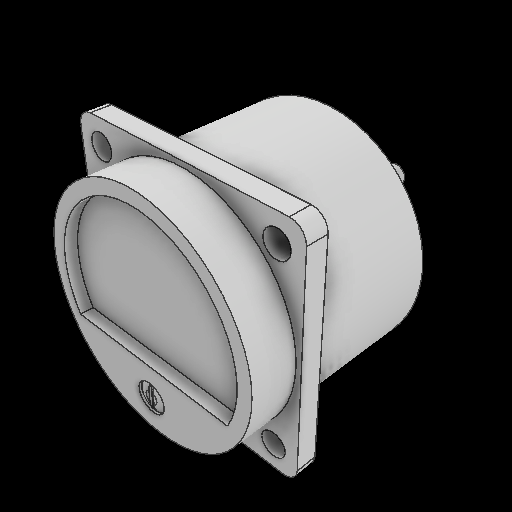
# Autodesk Inventor part: BaomanACPanelMountMeter
Saved by Autodesk Inventor 2025.2 (Build 292293000, 293)
## iProperties
Created: 2026-05-14
Part Number: BaomanACPanelMountMeter
Material: Generic
Document SubType Name: Modeling
Designer: valer
Density: 1 g/cm^3
Appearance: Default
Author: valer
Autodesk Inventor part; units mm, degrees
ref_plane "YZ Plane" through (0, 0, 0) normal (1, 0, 0) x (0, 1, 0)
ref_plane "XZ Plane" through (0, 0, 0) normal (0, 1, 0) x (-1, 0, 0)
ref_plane "XY Plane" through (0, 0, 0) normal (0, 0, 1) x (1, 0, 0)
sketch "Base" plane through (0, 0, 0) normal (0, 0, 1) x (1, 0, 0)
  line L0 (-23.5, -23.5) -> (23.5, -23.5)
  line L1 (23.5, -23.5) -> (23.5, 23.5)
  line L2 (23.5, 23.5) -> (-23.5, 23.5)
  line L3 (-23.5, 23.5) -> (-23.5, -23.5)
  line L4 (-23.5, -23.5) -> (23.5, 23.5) construction
  line L5 (23.5, -23.5) -> (-23.5, 23.5) construction
  point P0 (0, 0)
  dimension "d0" = 47
  constraints: 12 end point, 2 midpoint, 2 parallel, 2 perpendicular, 1 horizontal
  measures "d0" distance of L2.end L0.start
extrude "BaseFeature" add sketch "Base" along normal blind 4
fillet "FilletsFeature" radius 3 4 edges at (-23.5, -23.5, 2) (-23.5, 23.5, 2) (23.5, -23.5, 2) (23.5, 23.5, 2)
sketch "Front" plane through (0, 0, 4) normal (0, 0, 1) x (1, 0, 0)
  circle A0 centre (0, 0) radius 22.5
  dimension "d4" = 45
  constraints: 1 centre point, 1 coincident
  measures "d4" diameter of A0
extrude "FrontFeature" add sketch "Front" along normal blind 8.5
sketch "Screen" plane through (0, 0, 12.5) normal (0, 0, 1) x (1, 0, 0)
  circle A0 centre (0, 0) radius 19.7
  circle A1 centre (0, 0) radius 22.5 projected
  line L0 (-17.575, -8.9) -> (17.575, -8.9)
  line L1 (0, -8.9) -> (0, -19.7) construction
  dimension "d7" = 2.8
  dimension "d8" = 10.8
  constraints: 4 end point, 3 point on circle, 1 centre point, 1 coincident, 1 horizontal, 1 midpoint, 1 vertical
  measures "d7" radial gap between concentric circles of A1 A0
  measures "d8" distance of L1.start L1.end
extrude "ScreenFEature" cut sketch "Screen" against normal blind 2.5 contours A0 L0 picked at (4.7799, 0.8366)
sketch "ScrewHole" plane through (0, 0, 12.5) normal (0, 0, 1) x (1, 0, 0)
  line L0 (17.575, -8.9) -> (-17.575, -8.9) projected
  line L1 (0, -8.9) -> (0, -22.5) construction
  circle A0 centre (0, 0) radius 22.5 projected
  circle A1 centre (0, -15.7) radius 3
  circle A2 centre (0, -15.7) radius 3.1
  dimension "d11" = 6
  dimension "d12" = 0.1
  constraints: 2 centre point, 2 end point, 2 midpoint, 1 coincident, 1 vertical, 1 vertical alignment, 1 other
  measures "d11" diameter of A1
  measures "d12" radial gap between concentric circles of A2 A1
extrude "ScrewHoleFeature" cut sketch "ScrewHole" against normal blind 0.5 contours A1 | A2
sketch "ScrewHead" plane through (0, -15.7, 12) normal (0, 0, 1) x (1, 0, 0)
  circle A0 centre (0, 0) radius 3
  circle A1 centre (0, 0) radius 3.1 projected
  point P0 (0, 15.7)
  dimension "d15" = 6
  constraints: 1 centre point, 1 coincident
  measures "d15" diameter of A0
extrude "ScrewHeadFeature" add sketch "ScrewHead" along normal blind 0.5 contours A0
fillet "ScrewHeadFilletFeature" radius 3 1 edges at (-3, -15.7, 12.5)
sketch "ScrewFlat" plane through (0, -15.7, 12.5) normal (0, 0, 1) x (1, 0, 0)
  circle A0 centre (0, 0) radius 3 projected
  line L0 (0, 3) -> (0, -3) construction
  line L1 (-0.5, -2.5) -> (0.5, -2.5)
  line L2 (0.5, -2.5) -> (0.5, 2.5)
  line L3 (0.5, 2.5) -> (-0.5, 2.5)
  line L4 (-0.5, 2.5) -> (-0.5, -2.5)
  circle A1 centre (0, 0) radius 1.3417 projected
  line L5 (-0.5, -2.5) -> (0.5, 2.5) construction
  line L6 (0.5, -2.5) -> (-0.5, 2.5) construction
  point P0 (0, 15.7)
  dimension "d19" = 5
  dimension "d20" = 1
  constraints: 14 end point, 3 midpoint, 2 parallel, 2 point on circle, 1 horizontal, 1 perpendicular, 1 vertical
  measures "d19" distance of L1.end L2.end
  measures "d20" distance between parallel lines of L2 L4
extrude "ScrewFlatFeature" cut sketch "ScrewFlat" against normal blind 0.5 contours L4 A1 L2 L1 | L4 A1 L2 | L4 L3 L2 A1
sketch "MountHoles" plane through (0, 0, 4) normal (0, 0, 1) x (1, 0, 0)
  circle A0 centre (-18.5, -18.5) radius 2.5
  line L0 (-32.9, 0) -> (32.9, 0) projected
  line L1 (0, -32.9) -> (0, 32.9) projected
  circle A1 centre (18.5, -18.5) radius 2.5
  circle A2 centre (-18.5, 18.5) radius 2.5
  circle A3 centre (18.5, 18.5) radius 2.5
  point P0 (0, 0)
  dimension "d23" = 5
  dimension "d24" = 37
  dimension "d25" = 37
  constraints: 4 centre point, 3 symmetric about line, 3 other
  measures "d23" diameter of A0
  measures "d24" distance of A1.centre A0.centre
  measures "d25" distance of A0.centre A2.centre
extrude "MountHolesFeature" cut sketch "MountHoles" against normal through all
sketch "Body" plane through (0, 0, 0) normal (0, 0, -1) x (-1, 0, 0)
  circle A0 centre (0, 0) radius 22.5 projected
extrude "BodyFeature" add sketch "Body" along normal blind 25
sketch "Studs" plane through (0, 0, -25) normal (0, 0, -1) x (-1, 0, 0)
  circle A0 centre (0, 0) radius 22.5 projected
  line L0 (-21.2132, 7.5) -> (21.2132, 7.5) construction
  circle A1 centre (9.25, 9.5) radius 2
  line L1 (0, -32.9) -> (0, 32.9) construction
  circle A2 centre (-9.25, 9.5) radius 2
  line L2 (9.25, 9.5) -> (9.25, 7.5) construction
  line L3 (-9.25, 9.5) -> (-11.25, 9.5) construction
  line L4 (9.25, 9.5) -> (11.25, 9.5) construction
  point P0 (0, 22.5)
  dimension "d32" = 4
  dimension "d30" = 15
  dimension "d31" = 22.5
  constraints: 8 end point, 5 point on circle, 3 horizontal, 2 point on line, 1 centre point, 1 horizontal alignment, 1 symmetric about line, 1 vertical, 3 other
  measures "d30" distance from line of L0 point (0, 22.5)
  measures "d31" distance of L3.end L4.end
extrude "StudsFeature" add sketch "Studs" along normal blind 9 contours A1 | A2
equation "\"d25\" = d24"
body "Solid1"
